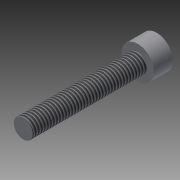
# Autodesk Inventor part: m5x0.8
Saved by Autodesk Inventor 2014 (Build 180170000, 170)
## iProperties
Created: 2014-10-05
Part Number: m5x0.8
Material: Generic
Document SubType Name: Modeling
Designer: Matthew
Density: 1 g/cm^3
Appearance: Default
Author: Matthew
Autodesk Inventor part; units mm, degrees
ref_plane "YZ Plane" through (0, 0, 0) normal (1, 0, 0) x (0, 1, 0)
ref_plane "XZ Plane" through (0, 0, 0) normal (0, 1, 0) x (-1, 0, 0)
ref_plane "XY Plane" through (0, 0, 0) normal (0, 0, 1) x (1, 0, 0)
sketch "Sketch1" plane through (0, 0, 0) normal (0, 0, 1) x (1, 0, 0)
  circle A0 centre (0, 0) radius 4.25
  dimension "d0" = 8.5
  constraints: 1 centre point, 1 coincident
  measures "d0" diameter of A0
extrude "Extrusion1" add sketch "Sketch1" along normal blind 5
sketch "Sketch2" plane through (0, 0, 5) normal (0, 0, 1) x (1, 0, 0)
  circle A0 centre (0, 0) radius 4.25 projected
  circle A1 centre (0, 0) radius 2.5
  dimension "d3" = 5
  constraints: 1 centre point, 1 coincident
  measures "d3" diameter of A1
extrude "Extrusion2" add sketch "Sketch2" along normal blind 30 contours A1
sketch "Sketch3" plane through (0, 0, 0) normal (0, 0, -1) x (-1, 0, 0)
  circle A0 centre (0, 0) radius 4.25 projected
  line L0 (2.3094, 0) -> (1.1547, -2)
  line L1 (1.1547, -2) -> (-1.1547, -2)
  line L2 (-1.1547, -2) -> (-2.3094, 0)
  line L3 (-2.3094, 0) -> (-1.1547, 2)
  line L4 (-1.1547, 2) -> (1.1547, 2)
  line L5 (1.1547, 2) -> (2.3094, 0)
  dimension "d6" = 4
  constraints: 12 end point, 1 coincident, 13 other
  measures "d6" distance between parallel lines of L1 L4
extrude "Extrusion3" cut sketch "Sketch3" against normal blind 3 contours L0 L1 L2 L3 L4 L5
thread "Thread1" size "M5x0.8" class "6g" standard "ANSI Metric M Profile" full length
body "Solid1"
